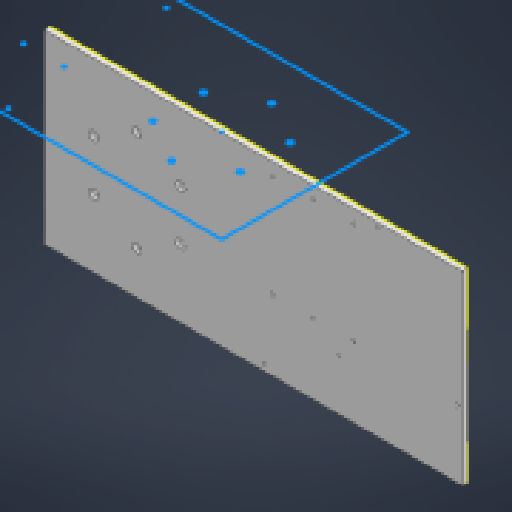
# Autodesk Inventor part: base plate
Saved by Autodesk Inventor 2026.2 (Build 302298000, 298)
## iProperties
Created: 2025-07-05
Part Number: base plate
Material: 一般
Document SubType Name: Modeling
Designer: gavin
Density: 1 g/cm^3
Appearance: 預設
Author: gavin
Autodesk Inventor part; units mm, degrees
ref_plane "YZ Plane" through (0, 0, 0) normal (1, 0, 0) x (0, 1, 0)
ref_plane "XZ Plane" through (0, 0, 0) normal (0, 1, 0) x (-1, 0, 0)
ref_plane "XY Plane" through (0, 0, 0) normal (0, 0, 1) x (1, 0, 0)
sketch "草圖1" plane through (0, 0, 0) normal (0, 0, 1) x (1, 0, 0)
  circle A0 centre (0, 0) radius 60 construction
  circle A1 centre (0, 0) radius 48 construction
  line L0 (350, -100) -> (-100, -100)
  line L1 (-100, -100) -> (-100, 100)
  line L2 (-100, 100) -> (350, 100)
  line L3 (350, 100) -> (350, -100)
  circle A2 centre (0, 54) radius 2.5
  circle A3 centre (-46.7654, 27) radius 2.5
  circle A4 centre (-46.7654, -27) radius 2.5
  circle A5 centre (0, -54) radius 2.5
  circle A6 centre (46.7654, -27) radius 2.5
  circle A7 centre (46.7654, 27) radius 2.5
  circle A8 centre (218.12, -44.54) radius 1.6 projected
  circle A9 centre (136.84, -92.8) radius 1.6 projected
  arc A10 (147.6, -24) -> (143.6, -24) centre (145.6, -24) ccw projected
  arc A11 (191.4, -24) -> (187.4, -24) centre (189.4, -24) ccw projected
  arc A12 (143.6, 86) -> (147.6, 86) centre (145.6, 86) ccw projected
  arc A13 (187.4, 86) -> (191.4, 86) centre (189.4, 86) ccw projected
  arc A14 (231.2, 86) -> (235.2, 86) centre (233.2, 86) ccw projected
  arc A15 (235.2, -24) -> (231.2, -24) centre (233.2, -24) ccw projected
  circle A16 centre (344.5, -27.5) radius 1.75 projected
  arc A17 (257.75, 95) -> (261.25, 95) centre (259.5, 95) ccw projected
  circle A18 centre (259.5, 95) radius 1.5
  circle A19 centre (233.2, 86) radius 1.5
  circle A20 centre (189.4, 86) radius 1.5
  circle A21 centre (145.6, 86) radius 1.5
  circle A22 centre (145.6, -24) radius 1.5
  circle A23 centre (189.4, -24) radius 1.5
  circle A24 centre (233.2, -24) radius 1.5
  circle A25 centre (218.12, -44.54) radius 1.5
  circle A26 centre (136.84, -92.8) radius 1.5
  circle A27 centre (344.5, -27.5) radius 1.5
  circle A28 centre (0, -54) radius 3.275 projected
  circle A29 centre (0, 54) radius 3.275 projected
  circle A30 centre (46.7654, -27) radius 3.275 projected
  circle A31 centre (-46.7654, -27) radius 3.275 projected
  circle A32 centre (-46.7654, 27) radius 3.275 projected
  circle A33 centre (46.7654, 27) radius 3.275 projected
  point P0 (0, 0)
  dimension "d0" = 450
  dimension "d1" = 200
  dimension "d2" = 100
  dimension "d3" = 100
  dimension "d6" = 5
  dimension "d9" = 360
  dimension "d14" = 3
  dimension "d15" = 3
  dimension "d16" = 3
  dimension "d17" = 3
  dimension "d18" = 3
  dimension "d19" = 3
  dimension "d20" = 3
  dimension "d21" = 3
  dimension "d22" = 3
  dimension "d23" = 3
  constraints: 16 centre point, 10 coincident, 8 end point, 2 parallel, 1 horizontal, 1 perpendicular, 13 other
  measures "d0" distance of L0.start L0.end
  measures "d1" distance of L2.end L0.start
  measures "d2" distance from line of point (0, 0) L1
  measures "d3" distance from line of L2 point (0, 0)
  measures "d6" diameter of A2
  measures "d14" diameter of A18
  measures "d15" diameter of A19
  measures "d16" diameter of A20
  measures "d17" diameter of A21
  measures "d18" diameter of A22
  measures "d19" diameter of A23
  measures "d20" diameter of A24
  measures "d21" diameter of A25
  measures "d22" diameter of A26
  measures "d23" diameter of A27
extrude "擠出1" add sketch "草圖1" along normal blind 6 contours L0 L1 L2 L3 | A28 | A29 | A30 | A31 | A32 | A33
chamfer "倒角1" distance 2.5 angle 45 6 edges at (-2.5, -54, 6) (-49.2654, -27, 6) (-49.2654, 27, 6) (-2.5, 54, 6) (44.2654, 27, 6) (44.2654, -27, 6)
sketch "草圖2" plane through (0, 0, 0) normal (0, 0, -1) x (-1, 0, 0)
  line L0 (-350, 100) -> (100, 100) projected
  line L1 (-350, -100) -> (-350, 100) projected
  line L2 (100, -100) -> (-350, -100) projected
  line L3 (100, 100) -> (100, -100) projected
  circle A0 centre (0, 54) radius 2.5 projected
  circle A1 centre (46.7654, 27) radius 2.5 projected
  circle A2 centre (46.7654, -27) radius 2.5 projected
  circle A3 centre (0, -54) radius 2.5 projected
  circle A4 centre (-46.7654, -27) radius 2.5 projected
  circle A5 centre (-46.7654, 27) radius 2.5 projected
  circle A6 centre (-233.2, -24) radius 1.5 projected
  circle A7 centre (-189.4, -24) radius 1.5 projected
  circle A8 centre (-145.6, -24) radius 1.5 projected
  circle A9 centre (-145.6, 86) radius 1.5 projected
  circle A10 centre (-189.4, 86) radius 1.5 projected
  circle A11 centre (-233.2, 86) radius 1.5 projected
  circle A12 centre (-259.5, 95) radius 1.5 projected
  circle A13 centre (-344.5, -27.5) radius 1.75 projected
  circle A14 centre (-136.84, -92.8) radius 1.6 projected
  circle A15 centre (-218.12, -44.54) radius 1.6 projected
  point P0 (0, 0)
